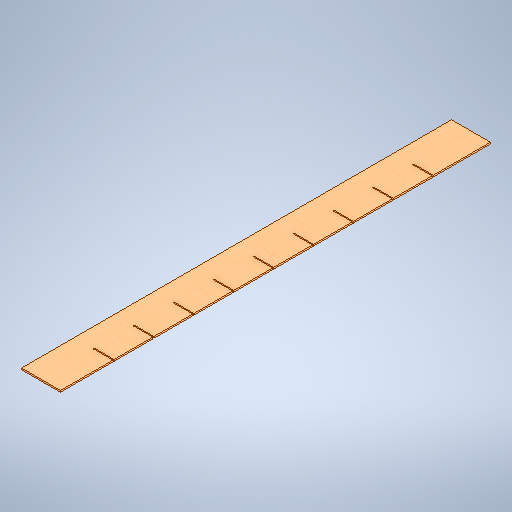
# Autodesk Inventor part: Base
Saved by Autodesk Inventor 2025.2 (Build 292293000, 293)
## iProperties
Created: 2025-05-12
Part Number: Base
Material: Wood (Cherry)
Document SubType Name: Modeling
Designer: USER
Density: 0.63 g/cm^3
Appearance: Cherry - Natural Low Gloss
Author: USER
Autodesk Inventor part; units mm, degrees
ref_plane "YZ Plane" through (0, 0, 0) normal (1, 0, 0) x (0, 1, 0)
ref_plane "XZ Plane" through (0, 0, 0) normal (0, 1, 0) x (-1, 0, 0)
ref_plane "XY Plane" through (0, 0, 0) normal (0, 0, 1) x (1, 0, 0)
sketch "Sketch1" plane through (0, 0, 0) normal (0, 1, 0) x (-1, 0, 0)
  line L0 (0, 0) -> (150, 0)
  line L1 (150, 0) -> (150, -1660)
  line L2 (150, -1660) -> (0, -1660)
  line L3 (0, -1660) -> (0, 0)
  dimension "d0" = 150
  dimension "d1" = 1660
  constraints: 8 end point, 2 parallel, 1 horizontal, 1 perpendicular
  measures "d0" distance of L1.end L2.end
  measures "d1" distance of L0.end L1.end
extrude "Extrusion1" add sketch "Sketch1" along normal blind 6
sketch "Sketch2" plane through (0, 6, 0) normal (0, 1, 0) x (1, 0, 0)
  line L0 (-150, 150) -> (0, 150)
  line L1 (-150, 0) -> (0, 0) projected
  line L2 (-150, 154) -> (0, 154)
  line L3 (-75, 150) -> (-75, 154)
  line L4 (-150, 304) -> (0, 304)
  line L5 (-150, 308) -> (0, 308)
  line L6 (-75, 304) -> (-75, 308)
  line L7 (-150, 458) -> (0, 458)
  line L8 (-150, 462) -> (0, 462)
  line L9 (-75, 458) -> (-75, 462)
  line L10 (-150, 612) -> (0, 612)
  line L11 (-150, 616) -> (0, 616)
  line L12 (-75, 612) -> (-75, 616)
  line L13 (-150, 766) -> (0, 766)
  line L14 (-150, 770) -> (0, 770)
  line L15 (-75, 766) -> (-75, 770)
  line L16 (-150, 920) -> (0, 920)
  line L17 (-150, 924) -> (0, 924)
  line L18 (-75, 920) -> (-75, 924)
  line L19 (-150, 1386) -> (0, 1386)
  line L20 (-150, 1382) -> (0, 1382)
  line L21 (-150, 1232) -> (0, 1232)
  line L22 (-150, 1228) -> (0, 1228)
  line L23 (-150, 1078) -> (0, 1078)
  line L24 (-150, 1074) -> (0, 1074)
  line L25 (-75, 1074) -> (-75, 1078)
  line L26 (-75, 1228) -> (-75, 1232)
  line L27 (-75, 1382) -> (-75, 1386)
  line L28 (0, 0) -> (0, 1660) projected
  line L29 (0, 0) -> (0, 1660)
  dimension "d4" = 150
  dimension "d5" = 4
  dimension "d6" = 150
  dimension "d7" = 4
  dimension "d8" = 150
  dimension "d9" = 4
  dimension "d10" = 150
  dimension "d11" = 4
  dimension "d12" = 150
  dimension "d13" = 4
  dimension "d14" = 150
  dimension "d15" = 4
  dimension "d19" = 150
  dimension "d21" = 150
  dimension "d22" = 150
  dimension "d40" = 4
  dimension "d41" = 4
  dimension "d42" = 4
  constraints: 56 end point, 18 midpoint, 3 horizontal, 2 vertical, 1 other
  measures "d4" distance between parallel lines of L0 L1
  measures "d5" distance between parallel lines of L0 L2
  measures "d6" distance between parallel lines of L4 L2
  measures "d7" distance between parallel lines of L4 L5
  measures "d8" distance between parallel lines of L7 L5
  measures "d9" distance from line of L9.end L7
  measures "d10" distance between parallel lines of L10 L8
  measures "d11" distance between parallel lines of L10 L11
  measures "d12" distance between parallel lines of L11 L13
  measures "d13" distance between parallel lines of L13 L14
  measures "d14" distance between parallel lines of L14 L16
  measures "d15" distance between parallel lines of L16 L17
  measures "d19" distance between parallel lines of L17 L24
  measures "d21" distance between parallel lines of L22 L23
  measures "d22" distance between parallel lines of L20 L21
  measures "d40" distance between parallel lines of L24 L23
  measures "d41" distance between parallel lines of L21 L22
  measures "d42" distance between parallel lines of L20 L19
extrude "Extrusion2" cut sketch "Sketch2" against normal blind 6
move faces "Move1" translate (0, 0, 53) faces at (-50, 2, -1660)
move faces "Move2" translate (0, 0, 53) faces at (-50, 4, 0)
body "Solid1"
